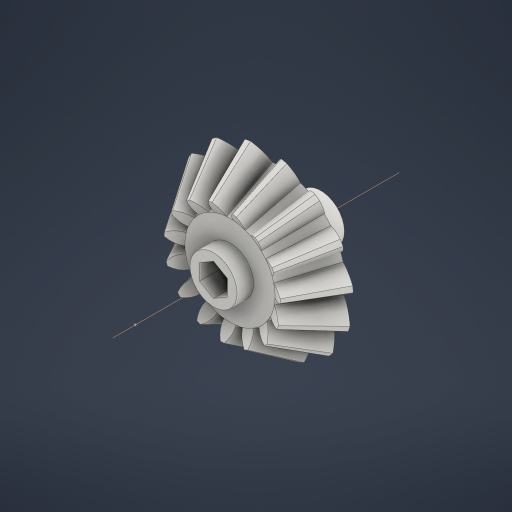
# Autodesk Inventor part: Bevel Gear2
Saved by Autodesk Inventor 2023 (Build 270158000, 158)
## iProperties
CustomPartVersion: 1
Created: 2022-11-09
Part Number: Bevel Gear2
Material: Steel, Mild
Document SubType Name: Modeling
Designer: izack
Categories: <?xml version="1.0" encoding="UTF-16"?> <MemberInstance><Categories><FamilyTemplate><FamilyTemplateParameter ValueType="xs:double" Id="1" ObjectReferenceKey="da_z" ObjectType="kUserParameterObject"/><FamilyTemplateParameter ValueType="xs:double" Id="2" ObjectReferenceKey="da_b" ObjectType="kUserParameterObject"/><FamilyTemplateParameter ValueType="xs:double" Id="3" ObjectReferenceKey="da_beta" ObjectType="kUserParameterObject"/><FamilyTemplateParameter ValueType="xs:double" Id="4" ObjectReferenceKey="da_dae" ObjectType="kUserParameterObject"/><FamilyTemplateParameter ValueType="xs:double" Id="5" ObjectReferenceKey="da_ve" ObjectType="kUserParameterObject"/><FamilyTemplateParameter ValueType="xs:double" Id="6" ObjectReferenceKey="da_omega" ObjectType="kUserParameterObject"/><FamilyTemplateParameter ValueType="xs:string" Id="7" ObjectReferenceKey="EAIAABAAAAAAHwAAAAAAAIAAAAAAAAAA" ObjectType="83914240" SubObjectId="SurfaceGeometry"/></FamilyTemplate><ParamToTemplateMap><ParamToTemplate CategoryParameter="//CategoryParameter[@InternalName='046C89C9-8512-4d59-83FE-43B91F4F132A']" TemplateParameter="1"/><ParamToTemplate CategoryParameter="//CategoryParameter[@InternalName='2552DF32-E462-4b46-AEBF-C6C7768E72AC']" TemplateParameter="2"/><ParamToTemplate CategoryParameter="//CategoryParameter[@InternalName='C9EE641D-15FC-4fae-A226-E94C4372FDD7']" TemplateParameter="3"/><ParamToTemplate><ParamToTemplate CategoryParameter="//CategoryParameter[@InternalName='00B6519A-459B-49c7-AD84-2E56D39A5744']" ConstantValue="-0.000000"/></ParamToTemplate><ParamToTemplate><ParamToTemplate CategoryParameter="//CategoryParameter[@InternalName='04B31F0E-C7A6-4894-AA32-9629BEFACF47']" ConstantValue="1.000000"/></ParamToTemplate><ParamToTemplate><ParamToTemplate CategoryParameter="//CategoryParameter[@InternalName='43CBEC2E-7847-49e7-A936-2F7889FCB2D9']" ConstantValue="0.200000"/></ParamToTemplate><ParamToTemplate><ParamToTemplate CategoryParameter="//CategoryParameter[@InternalName='B1EFC894-105D-4ebd-86BF-FA20ED196853']" ConstantValue="0.300000"/></ParamToTemplate><ParamToTemplate><ParamToTemplate CategoryParameter="//CategoryParameter[@InternalName='51175063-3D10-4879-93E8-6246FE8B403D']" ConstantValue="2060000000.000000"/></ParamToTemplate><ParamToTemplate><ParamToTemplate CategoryParameter="//CategoryParameter[@InternalName='A3A52E27-4454-46a9-B0BD-C932399B70AF']" ConstantValue="0.300000"/></ParamToTemplate><ParamToTemplate CategoryParameter="//CategoryParameter[@InternalName='2A200944-5A8C-41ca-B96E-8520D2E510F1']" TemplateParameter="4"/><ParamToTemplate><ParamToTemplate CategoryParameter="//CategoryParameter[@InternalName='1A637F62-92C8-44bc-B81F-10802510B579']" ConstantValue="2.231602"/></ParamToTemplate><ParamToTemplate CategoryParameter="//CategoryParameter[@InternalName='B52DD4BE-6863-48fb-BF58-89EF6F9EC65C']" TemplateParameter="5"/><ParamToTemplate><ParamToTemplate CategoryParameter="//CategoryParameter[@InternalName='3956BFF2-84D2-457d-93C2-9B0613DEBA67']" ConstantValue="1.667166"/></ParamToTemplate><ParamToTemplate CategoryParameter="//CategoryParameter[@InternalName='739CFA02-461B-4bf8-8049-181FCAD8B28F']" TemplateParameter="6"/><ParamToTemplate><ParamToTemplate CategoryParameter="//CategoryParameter[@InternalName='A27E999F-E2CE-4481-8A2A-EBF499C4C3C5']" ConstantValue="-0.000000"/></ParamToTemplate><ParamToTemplate><ParamToTemplate CategoryParameter="//CategoryParameter[@InternalName='9E1B4470-B2D3-4ff1-B813-535BB4CDF51A']" ConstantValue="3520000.000000"/></ParamToTemplate><ParamToTemplate><ParamToTemplate CategoryParameter="//CategoryParameter[@InternalName='F8452263-BFF6-458c-9FB1-07C4B99E95CD']" ConstantValue="11400000.000000"/></ParamToTemplate><ParamToTemplate><ParamToTemplate CategoryParameter="//CategoryParameter[@InternalName='3E3BB259-FD49-497f-8171-6EBC954A3479']" ConstantValue="2.000000"/></ParamToTemplate><ParamToTemplate CategoryParameter="//CategoryParameter[@InternalName='27C3BAF2-7550-4e4b-AE2C-0DB134B7D9B7']" TemplateParameter="7"/></ParamToTemplateMap><Category DisplayName="Gear" InternalName="DC85795E-93AB-48d5-8EEE-5A27447B64BD" Mnemonic="Gear"><CategoryParameter DisplayName="z" InternalName="046C89C9-8512-4d59-83FE-43B91F4F132A" Mnemonic="z"/><CategoryParameter DisplayName="b" InternalName="2552DF32-E462-4b46-AEBF-C6C7768E72AC" Mnemonic="b"/><CategoryParameter DisplayName="||b|" InternalName="C9EE641D-15FC-4fae-A226-E94C4372FDD7" Mnemonic="beta"/><CategoryParameter DisplayName="x" InternalName="00B6519A-459B-49c7-AD84-2E56D39A5744" Mnemonic="x"/><CategoryParameter DisplayName="a*" InternalName="04B31F0E-C7A6-4894-AA32-9629BEFACF47" Mnemonic="a"/><CategoryParameter DisplayName="c*" InternalName="43CBEC2E-7847-49e7-A936-2F7889FCB2D9" Mnemonic="c"/><CategoryParameter DisplayName="r|.f|*" InternalName="B1EFC894-105D-4ebd-86BF-FA20ED196853" Mnemonic="rf"/><CategoryParameter DisplayName="E" InternalName="51175063-3D10-4879-93E8-6246FE8B403D" Mnemonic="E"/><CategoryParameter DisplayName="||m|" InternalName="A3A52E27-4454-46a9-B0BD-C932399B70AF" Mnemonic="mi"/><Category DisplayName="BevelGear" InternalName="0C98F69A-0C2B-4791-B2FE-7691BB227E77" Mnemonic="BevelGear"><CategoryParameter DisplayName="d|.ae|" InternalName="2A200944-5A8C-41ca-B96E-8520D2E510F1" Mnemonic="dae"/><CategoryParameter DisplayName="d|.ai|" InternalName="1A637F62-92C8-44bc-B81F-10802510B579" Mnemonic="dai"/><CategoryParameter DisplayName="A|.e|" InternalName="B52DD4BE-6863-48fb-BF58-89EF6F9EC65C" Mnemonic="ve"/><CategoryParameter DisplayName="A|.i|" InternalName="3956BFF2-84D2-457d-93C2-9B0613DEBA67" Mnemonic="vi"/><CategoryParameter DisplayName="||S|" InternalName="739CFA02-461B-4bf8-8049-181FCAD8B28F" Mnemonic="omega"/><CategoryParameter DisplayName="x|.t|" InternalName="A27E999F-E2CE-4481-8A2A-EBF499C4C3C5" Mnemonic="xt"/><CategoryParameter DisplayName="||s||.Flim|" InternalName="9E1B4470-B2D3-4ff1-B813-535BB4CDF51A" Mnemonic="sFlim"/><CategoryParameter DisplayName="||s||.Hlim|" InternalName="F8452263-BFF6-458c-9FB1-07C4B99E95CD" Mnemonic="sHlim"/><CategoryParameter DisplayName="type" InternalName="3E3BB259-FD49-497f-8171-6EBC954A3479" Mnemonic="type"/><CategoryParameter DisplayName="PitchDiameter" InternalName="27C3BAF2-7550-4e4b-AE2C-0DB134B7D9B7" Mnemonic="IDS_PITCHDIAM"/></Category></Category></Categories></MemberInstance>
Mass: 60.9118 g
Surface Area: 34.3074 cm^2
Volume: 7.7496 cm^3
Density: 7.86 g/cm^3
Appearance: Steel
Author: izack
## iProperties of the stored document Bevel Gear21_3DPrint.ipt
Part Number: Bevel Gear21_3DPrint
Material: Generic
Document SubType Name: Modeling
Designer: izack
Appearance: Default
Author: izack
Autodesk Inventor part; units mm, degrees
ref_plane "Mesh Plane2" through (0, 0, 0) normal (0.9781476, 0.2079117, 0) x (0, 0, 1)
sketch "Teeth Body Sketch" plane through (0, 0, 0) normal (1, 0, 0) x (0, 1, 0)
  line L0 (0, 0) -> (12.921155, -27.199334) construction
  line L1 (12.921155, -27.199334) -> (16.732371, -25.000555)
  line L2 (16.732371, -25.000555) -> (0, 0) construction
  line L3 (15, -26) -> (0, 0) construction
  line L4 (8.616494, -18.137922) -> (11.15801, -16.671663)
  line L5 (12.921155, -27.199334) -> (8.616494, -18.137922)
  line L6 (16.732371, -25.000555) -> (11.15801, -16.671663)
  line L7 (0, -41.235694) -> (0, 6.872616)
  line L8 (0, -26) -> (16.732371, -26) construction
  dimension "d0" = 30
  dimension "d1" = 25.84231
  dimension "d2" = 33.46474
  dimension "d3" = 10
  dimension "d4" = 25.00056
  constraints: 16 end point, 4 point on line, 3 perpendicular, 2 collinear, 1 horizontal alignment, 1 vertical alignment
  measures "d0" diameter of L3.start L7
  measures "d1" diameter of L0.end L7
  measures "d2" diameter of L1.end L7
  measures "d3" distance between parallel lines of L1 L4
  measures "d4" vertical distance of L1.end L0.start
revolve "Teeth Body" add sketch "Teeth Body Sketch" angle 360 about axis through (0, 0, 0) along (0, 0, 1)
ref_plane "Tooth Plane" through (0, 15, -26) normal (0, -0.4997225, 0.8661856) x (1, 0, 0)
sketch "Start Sketch" plane through (0, 15, -26) normal (0, -0.4997225, 0.8661856) x (1, 0, 0)
  line L0 (0, -22.868969) -> (0, 9.184086)
  arc A0 (-0.903707, -2.928) -> (-4.426253, 2.839745) centre (-7.495058, -2.99401) ccw
  arc A1 (4.426253, 2.839745) -> (0.903707, -2.928) centre (7.495058, -2.99401) ccw
  line L1 (-0.903707, -2.928) -> (0.903707, -2.928)
  arc A2 (4.426253, 2.839745) -> (-4.426253, 2.839745) centre (0, -17.317305) ccw
  dimension "d7" = 6.59168
  dimension "d8" = 7.49506
  dimension "d9" = 14.32329
  dimension "d57" = 20.63731
  dimension "d58" = 14.38931
  constraints: 6 point on circle, 3 centre point, 3 symmetric about line, 2 end point, 1 coincident, 1 perpendicular, 1 other
  measures "d7" radius of A0
  measures "d8" horizontal distance of point (0, -17.317) A0.centre
  measures "d9" vertical distance of point (0, -17.317) A0.centre
  measures "d57" radius of A2
  measures "d58" distance from line of A2.centre L1
sketch "End Sketch" plane through (0, 9.892837, -17.147583) normal (0, -0.4997225, 0.8661856) x (1, 0, 0)
  line L0 (0, -19.092274) -> (0, 7.667381)
  arc A0 (-0.596015, -1.931082) -> (-2.919213, 1.872875) centre (-4.943159, -1.974617) ccw
  arc A1 (2.919213, 1.872875) -> (0.596015, -1.931082) centre (4.943159, -1.974617) ccw
  line L1 (-0.596015, -1.931082) -> (0.596015, -1.931082)
  arc A2 (2.919213, 1.872875) -> (-2.919213, 1.872875) centre (0, -11.421151) ccw
  dimension "d12" = 4.34736
  dimension "d15" = 4.94316
  dimension "d16" = 9.44653
  dimension "d59" = 13.61077
  dimension "d60" = 9.49007
  constraints: 6 point on circle, 3 centre point, 3 symmetric about line, 2 end point, 1 coincident, 1 other
  measures "d12" radius of A0
  measures "d15" horizontal distance of A0.centre point (0, -11.421)
  measures "d16" vertical distance of A0.centre point (0, -11.421)
  measures "d59" radius of A2
  measures "d60" distance from line of A2.centre L1
loft "Loft" cut profiles "Start Sketch", "End Sketch"
pattern_circular "Circular Pattern" count 15 over 360 about axis through (0, 0, 0) along (0, 0, 1) of "Loft"
ref_plane "End Plane" through (0, 9.892837, -17.147583) normal (0, -0.4997225, 0.8661856) x (1, 0, 0)
sketch3d "3D Sketch Right"
ref_plane "End Plane Right" through (-2.302354, 9.621194, -17.147583) normal (0.1163001, -0.4860008, 0.8661856) x (0.9725415, 0.2327294, 0)
sketch "End Sketch Right" plane through (-2.302354, 9.621194, -17.147583) normal (0.1163001, -0.4860008, 0.8661856) x (0.9725415, 0.2327294, 0)
  arc A0 (-0.596015, -1.931082) -> (-2.919213, 1.872875) centre (-4.943159, -1.974617) ccw
  line L0 (0, -22.925623) -> (0, 11.500729)
  arc A1 (2.919213, 1.872875) -> (0.596015, -1.931082) centre (4.943159, -1.974617) ccw
  line L1 (-0.596015, -1.931082) -> (0.596015, -1.931082)
  arc A2 (2.919213, 1.872875) -> (-2.919213, 1.872875) centre (0, -11.421151) ccw
  dimension "d70" = 4.94316
  dimension "d71" = 9.44653
  dimension "d72" = 4.34736
  dimension "d73" = 9.49007
  dimension "d74" = 13.61077
  constraints: 6 point on circle, 3 centre point, 3 symmetric about line, 2 end point, 1 coincident, 1 perpendicular, 1 other
  measures "d70" horizontal distance of A2.centre A0.centre
  measures "d71" vertical distance of point (0, -11.421) A0.centre
  measures "d72" radius of A0
  measures "d73" distance from line of point (0, -11.421) L1
  measures "d74" radius of A2
feature "Loft Right" [suppressed]
pattern_circular "Circular Pattern Right" [suppressed]
sketch3d "3D Sketch Left"
ref_plane "End Plane Left" through (2.284511, 9.621194, -17.142962) normal (-0.1154342, -0.4861499, 0.8662178) x (0.9729484, -0.2310224, 0)
sketch "End Sketch Left" plane through (2.284511, 9.621194, -17.142962) normal (-0.1154342, -0.4861499, 0.8662178) x (0.9729484, -0.2310224, 0)
  line L0 (0, -32.441688) -> (0, 15.485439)
  arc A0 (-0.596015, -1.929807) -> (-2.919213, 1.87415) centre (-4.943159, -1.973342) ccw
  arc A1 (2.919213, 1.87415) -> (0.596015, -1.929807) centre (4.943159, -1.973342) ccw
  line L1 (-0.596015, -1.929807) -> (0.596015, -1.929807)
  ellipse E0 centre (0, -8.330274) end of major axis (11.15801, -8.330274) minor radius 9.665267
  arc A2 (2.919213, 1.87415) -> (-2.919213, 1.87415) centre (0, -11.419876) ccw
  dimension "d56" = 9.66527
  dimension "d30" = 4.34736
  dimension "d31" = 4.94316
  dimension "d32" = 9.44653
  dimension "d61" = 13.61077
  dimension "d62" = 9.49007
  constraints: 6 point on circle, 3 centre point, 3 symmetric about line, 2 end point, 1 coincident, 2 other
  measures "d30" radius of A0
  measures "d31" horizontal distance of point (0, -11.42) A0.centre
  measures "d32" vertical distance of A0.centre point (0, -11.42)
  measures "d61" radius of A2
  measures "d62" distance from line of point (0, -11.42) L1
feature "Loft Left" [suppressed]
pattern_circular "Circular Pattern Left" [suppressed]
sketch "Body Sketch" plane through (0, 0, 0) normal (1, 0, 0) x (0, 1, 0)
  line L0 (0, -35.905122) -> (0, -25.110819)
  line L1 (12.921155, -27.199334) -> (8.616494, -18.137922)
  line L2 (8.616494, -18.137922) -> (0, -18.137922)
  line L3 (12.921155, -27.199334) -> (0, -27.199334)
  constraints: 4 end point, 2 perpendicular, 2 point on line
sketch "Body Sketch outline for Fix Body" plane through (0, 0, 0) normal (1, 0, 0) x (0, 1, 0)
  line L0 (0, -27.199334) -> (12.921155, -27.199334)
  line L1 (0, -18.137922) -> (0, -27.199334)
  line L2 (8.616494, -18.137922) -> (0, -18.137922)
  line L3 (12.921155, -27.199334) -> (8.616494, -18.137922)
revolve "Fix Body" add sketch "Body Sketch outline for Fix Body" angle 360 about axis through (0, 0, 0) along (0, 0, 1)
sketch "Sketch6" plane through (0, 0, 0) normal (1, 0, 0) x (0, 1, 0)
  line L0 (15, -26) -> (0, 0) projected
  line L1 (0, -39.6) -> (0, 6.6) projected
surface revolve "Pitch Diameter" sketch "Sketch6" angle 360 about axis through (0, 0, 0) along (0, 0, 1) shown no curves L0
sketch "Sketch8" plane through (0, 0, -18.137922) normal (0, 0, 1) x (1, 0, 0)
  circle A0 centre (0, 0) radius 2.65
  line L0 (-2.65, 1.529978) -> (0, 3.059956)
  line L1 (0, 3.059956) -> (2.65, 1.529978)
  line L2 (2.65, 1.529978) -> (2.65, -1.529978)
  line L3 (2.65, -1.529978) -> (0, -3.059956)
  line L4 (0, -3.059956) -> (-2.65, -1.529978)
  line L5 (-2.65, -1.529978) -> (-2.65, 1.529978)
  circle A1 centre (0, 0) radius 4.5
  point P0 (-2.65, 0)
  dimension "d94" = 5.3
  dimension "d95" = 9
  constraints: 12 end point, 3 coincident, 1 centre point, 1 horizontal alignment, 1 midpoint, 15 other
  measures "d95" diameter of A1
extrude "Extrusion1" cut sketch "Sketch8" against normal through all contours A0 | L2 L3 A0 | A0 L1 L2 | A0 L0 L1 | L3 L4 A0 | A0 L5 L0 | L4 L5 A0
ref_plane "Work Plane6" through (-7.585705, -7.585705, -15) normal (0, 0, -1) x (-0.1795152, 0.9837552, 0)
ref_plane "Work Plane7" through (-8.24961, -8.24961, -48) normal (0, 0, 1) x (0.9625177, 0.2712187, 0)
ref_plane "Work Plane8" through (-18.478937, -25.874651, -35.5) normal (0, 0, 1) x (0.8202519, 0.5720024, 0)
ref_plane "Work Plane9" through (-4.606756, -4.606756, -15) normal (0, 0, -1) x (-0.2337376, 0.9722997, 0)
extrude "Extrusion2" add sketch "Sketch8" along normal up to surface (20.5 mm away) from surface at -17.362078
equation "\"d0\" = da_de"
equation "\"d1\" = da_dfe"
equation "\"d2\" = da_dae"
equation "\"d3\" = da_b"
equation "\"d4\" = da_ve"
equation "\"d7\" = fd_rr"
equation "\"d8\" = fd_x"
equation "\"d9\" = fd_y"
equation "\"d57\" = 0.5 * fd_dva + 0.3 * da_he"
equation "\"d58\" = 0.5 * fd_dva - 1.12 * da_he"
equation "\"da_teethtype\" = 0"
equation "\"da_b\" = 10"
equation "\"da_de\" = 30"
equation "\"da_dae\" = 33.46474"
equation "\"da_dfe\" = 25.84231"
equation "\"da_le\" = 30.01666"
equation "\"da_omega\" = 90deg"
equation "\"da_beta\" = 0"
equation "\"da_delta\" = 29.981639deg"
equation "\"da_alpha\" = 20deg"
equation "\"da_he\" = 4.4"
equation "\"da_ve\" = 25.00056"
equation "\"da_zv\" = 17.317305"
equation "\"fd_loft\" = da_b + 0.05 * da_he"
equation "\"fd_x\" = fd_x1 + fd_x2"
equation "\"fd_y\" = fd_y1 - fd_y2"
equation "\"fd_dd\" = fd_dva - 0.8 * da_he"
equation "\"da_dvw\" = 34.63461"
equation "\"d11\" = fd_loft"
equation "\"da_dm\" = 25.00278"
equation "\"da_x\" = 0"
equation "\"da_m\" = 2"
equation "\"d50\" = da_omega"
equation "\"fd_rr\" = 6.591681"
equation "\"fd_dva\" = 38.63461"
equation "\"fd_x1\" = 1.586024"
equation "\"fd_x2\" = 5.909034"
equation "\"fd_y1\" = 17.244523"
equation "\"fd_y2\" = 2.921229"
body "Solid1"
body "Srf1"
